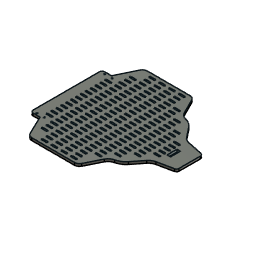
Electronics plate v13 (Autodesk Fusion 360 design; units mm, degrees)
Autodesk Fusion 360 part; units mm, degrees
(part 1 of 4)
sketch "Sketch2" plane through (0, 0, 0) normal (0, 1, 0) x (1, 0, 0)
  line L0 (-228.4396, 191.0218) -> (-250, 146.0218)
  line L1 (-249.9865, 0) -> (-228.4396, -44.9718)
  line L2 (-128.4396, 191.0218) -> (-228.4396, 191.0218)
  line L3 (-228.4396, -44.9718) -> (-128.4396, -44.9718)
  line L4 (-105.9194, 146.05) -> (-128.4396, 191.0218)
  line L5 (-128.4396, -44.9718) -> (-105.9194, 0)
  line L6 (-138.6977, 71.525) -> (-143.6977, 71.525)
  line L7 (-148.6977, 74.525) -> (-138.6977, 74.525)
  arc A0 (-138.6977, 71.525) -> (-138.6977, 74.525) centre (-138.6977, 73.025) ccw
  arc A1 (-148.6977, 74.525) -> (-148.6977, 71.525) centre (-148.6977, 73.025) ccw
  line L8 (-148.6977, 71.525) -> (-143.6977, 71.525)
  arc A2 (-208.6977, -35.475) -> (-208.6977, -38.475) centre (-208.6977, -36.975) ccw
  arc A3 (-198.6977, -38.475) -> (-198.6977, -35.475) centre (-198.6977, -36.975) ccw
  line L9 (-208.6977, -35.475) -> (-198.6977, -35.475)
  line L10 (-208.6977, -38.475) -> (-203.6977, -38.475)
  line L11 (-198.6977, -38.475) -> (-203.6977, -38.475)
  arc A4 (-188.6977, -35.475) -> (-188.6977, -38.475) centre (-188.6977, -36.975) ccw
  arc A5 (-178.6977, -38.475) -> (-178.6977, -35.475) centre (-178.6977, -36.975) ccw
  line L12 (-188.6977, -35.475) -> (-178.6977, -35.475)
  line L13 (-188.6977, -38.475) -> (-183.6977, -38.475)
  line L14 (-178.6977, -38.475) -> (-183.6977, -38.475)
  arc A6 (-168.6977, -35.475) -> (-168.6977, -38.475) centre (-168.6977, -36.975) ccw
  arc A7 (-158.6977, -38.475) -> (-158.6977, -35.475) centre (-158.6977, -36.975) ccw
  line L15 (-168.6977, -35.475) -> (-158.6977, -35.475)
  line L16 (-168.6977, -38.475) -> (-163.6977, -38.475)
  line L17 (-158.6977, -38.475) -> (-163.6977, -38.475)
  arc A8 (-148.6977, -35.475) -> (-148.6977, -38.475) centre (-148.6977, -36.975) ccw
  arc A9 (-138.6977, -38.475) -> (-138.6977, -35.475) centre (-138.6977, -36.975) ccw
  line L18 (-148.6977, -35.475) -> (-138.6977, -35.475)
  line L19 (-148.6977, -38.475) -> (-143.6977, -38.475)
  line L20 (-138.6977, -38.475) -> (-143.6977, -38.475)
  arc A10 (-208.6977, -25.475) -> (-208.6977, -28.475) centre (-208.6977, -26.975) ccw
  arc A11 (-198.6977, -28.475) -> (-198.6977, -25.475) centre (-198.6977, -26.975) ccw
  line L21 (-208.6977, -25.475) -> (-198.6977, -25.475)
  line L22 (-208.6977, -28.475) -> (-203.6977, -28.475)
  line L23 (-198.6977, -28.475) -> (-203.6977, -28.475)
  arc A12 (-188.6977, -25.475) -> (-188.6977, -28.475) centre (-188.6977, -26.975) ccw
  arc A13 (-178.6977, -28.475) -> (-178.6977, -25.475) centre (-178.6977, -26.975) ccw
  line L24 (-188.6977, -25.475) -> (-178.6977, -25.475)
  line L25 (-188.6977, -28.475) -> (-183.6977, -28.475)
  line L26 (-178.6977, -28.475) -> (-183.6977, -28.475)
  arc A14 (-168.6977, -25.475) -> (-168.6977, -28.475) centre (-168.6977, -26.975) ccw
  arc A15 (-158.6977, -28.475) -> (-158.6977, -25.475) centre (-158.6977, -26.975) ccw
  line L27 (-168.6977, -25.475) -> (-158.6977, -25.475)
  line L28 (-168.6977, -28.475) -> (-163.6977, -28.475)
  line L29 (-158.6977, -28.475) -> (-163.6977, -28.475)
  arc A16 (-148.6977, -25.475) -> (-148.6977, -28.475) centre (-148.6977, -26.975) ccw
  arc A17 (-138.6977, -28.475) -> (-138.6977, -25.475) centre (-138.6977, -26.975) ccw
  line L30 (-148.6977, -25.475) -> (-138.6977, -25.475)
  line L31 (-148.6977, -28.475) -> (-143.6977, -28.475)
  line L32 (-138.6977, -28.475) -> (-143.6977, -28.475)
  arc A18 (-228.6977, -15.475) -> (-228.6977, -18.475) centre (-228.6977, -16.975) ccw
  arc A19 (-218.6977, -18.475) -> (-218.6977, -15.475) centre (-218.6977, -16.975) ccw
  line L33 (-228.6977, -15.475) -> (-218.6977, -15.475)
  line L34 (-228.6977, -18.475) -> (-223.6977, -18.475)
  line L35 (-218.6977, -18.475) -> (-223.6977, -18.475)
  arc A20 (-208.6977, -15.475) -> (-208.6977, -18.475) centre (-208.6977, -16.975) ccw
  arc A21 (-198.6977, -18.475) -> (-198.6977, -15.475) centre (-198.6977, -16.975) ccw
  line L36 (-208.6977, -15.475) -> (-198.6977, -15.475)
  line L37 (-208.6977, -18.475) -> (-203.6977, -18.475)
  line L38 (-198.6977, -18.475) -> (-203.6977, -18.475)
  arc A22 (-188.6977, -15.475) -> (-188.6977, -18.475) centre (-188.6977, -16.975) ccw
  arc A23 (-178.6977, -18.475) -> (-178.6977, -15.475) centre (-178.6977, -16.975) ccw
  line L39 (-188.6977, -15.475) -> (-178.6977, -15.475)
  line L40 (-188.6977, -18.475) -> (-183.6977, -18.475)
  line L41 (-178.6977, -18.475) -> (-183.6977, -18.475)
  arc A24 (-168.6977, -15.475) -> (-168.6977, -18.475) centre (-168.6977, -16.975) ccw
  arc A25 (-158.6977, -18.475) -> (-158.6977, -15.475) centre (-158.6977, -16.975) ccw
  line L42 (-168.6977, -15.475) -> (-158.6977, -15.475)
  line L43 (-168.6977, -18.475) -> (-163.6977, -18.475)
  line L44 (-158.6977, -18.475) -> (-163.6977, -18.475)
  arc A26 (-148.6977, -15.475) -> (-148.6977, -18.475) centre (-148.6977, -16.975) ccw
  arc A27 (-138.6977, -18.475) -> (-138.6977, -15.475) centre (-138.6977, -16.975) ccw
  line L45 (-148.6977, -15.475) -> (-138.6977, -15.475)
  line L46 (-148.6977, -18.475) -> (-143.6977, -18.475)
  line L47 (-138.6977, -18.475) -> (-143.6977, -18.475)
  arc A28 (-228.6977, -5.475) -> (-228.6977, -8.475) centre (-228.6977, -6.975) ccw
  arc A29 (-218.6977, -8.475) -> (-218.6977, -5.475) centre (-218.6977, -6.975) ccw
  line L48 (-228.6977, -5.475) -> (-218.6977, -5.475)
  line L49 (-228.6977, -8.475) -> (-223.6977, -8.475)
  line L50 (-218.6977, -8.475) -> (-223.6977, -8.475)
  arc A30 (-208.6977, -5.475) -> (-208.6977, -8.475) centre (-208.6977, -6.975) ccw
  arc A31 (-198.6977, -8.475) -> (-198.6977, -5.475) centre (-198.6977, -6.975) ccw
  line L51 (-208.6977, -5.475) -> (-198.6977, -5.475)
  line L52 (-208.6977, -8.475) -> (-203.6977, -8.475)
  line L53 (-198.6977, -8.475) -> (-203.6977, -8.475)
  arc A32 (-188.6977, -5.475) -> (-188.6977, -8.475) centre (-188.6977, -6.975) ccw
  arc A33 (-178.6977, -8.475) -> (-178.6977, -5.475) centre (-178.6977, -6.975) ccw
  line L54 (-188.6977, -5.475) -> (-178.6977, -5.475)
  line L55 (-188.6977, -8.475) -> (-183.6977, -8.475)
  line L56 (-178.6977, -8.475) -> (-183.6977, -8.475)
  arc A34 (-168.6977, -5.475) -> (-168.6977, -8.475) centre (-168.6977, -6.975) ccw
  arc A35 (-158.6977, -8.475) -> (-158.6977, -5.475) centre (-158.6977, -6.975) ccw
  line L57 (-168.6977, -5.475) -> (-158.6977, -5.475)
  line L58 (-168.6977, -8.475) -> (-163.6977, -8.475)
  line L59 (-158.6977, -8.475) -> (-163.6977, -8.475)
  arc A36 (-148.6977, -5.475) -> (-148.6977, -8.475) centre (-148.6977, -6.975) ccw
  arc A37 (-138.6977, -8.475) -> (-138.6977, -5.475) centre (-138.6977, -6.975) ccw
  line L60 (-148.6977, -5.475) -> (-138.6977, -5.475)
  line L61 (-148.6977, -8.475) -> (-143.6977, -8.475)
  line L62 (-138.6977, -8.475) -> (-143.6977, -8.475)
  arc A38 (-128.6977, -5.475) -> (-128.6977, -8.475) centre (-128.6977, -6.975) ccw
  arc A39 (-118.6977, -8.475) -> (-118.6977, -5.475) centre (-118.6977, -6.975) ccw
  line L63 (-128.6977, -5.475) -> (-118.6977, -5.475)
  line L64 (-128.6977, -8.475) -> (-123.6977, -8.475)
  line L65 (-118.6977, -8.475) -> (-123.6977, -8.475)
  arc A40 (-228.6977, 4.525) -> (-228.6977, 1.525) centre (-228.6977, 3.025) ccw
  arc A41 (-218.6977, 1.525) -> (-218.6977, 4.525) centre (-218.6977, 3.025) ccw
  line L66 (-228.6977, 4.525) -> (-218.6977, 4.525)
  line L67 (-228.6977, 1.525) -> (-223.6977, 1.525)
  line L68 (-218.6977, 1.525) -> (-223.6977, 1.525)
  arc A42 (-208.6977, 4.525) -> (-208.6977, 1.525) centre (-208.6977, 3.025) ccw
  arc A43 (-198.6977, 1.525) -> (-198.6977, 4.525) centre (-198.6977, 3.025) ccw
  line L69 (-208.6977, 4.525) -> (-198.6977, 4.525)
  line L70 (-208.6977, 1.525) -> (-203.6977, 1.525)
  line L71 (-198.6977, 1.525) -> (-203.6977, 1.525)
  arc A44 (-188.6977, 4.525) -> (-188.6977, 1.525) centre (-188.6977, 3.025) ccw
  arc A45 (-178.6977, 1.525) -> (-178.6977, 4.525) centre (-178.6977, 3.025) ccw
  line L72 (-188.6977, 4.525) -> (-178.6977, 4.525)
  line L73 (-188.6977, 1.525) -> (-183.6977, 1.525)
  line L74 (-178.6977, 1.525) -> (-183.6977, 1.525)
  arc A46 (-168.6977, 4.525) -> (-168.6977, 1.525) centre (-168.6977, 3.025) ccw
  arc A47 (-158.6977, 1.525) -> (-158.6977, 4.525) centre (-158.6977, 3.025) ccw
  line L75 (-168.6977, 4.525) -> (-158.6977, 4.525)
  line L76 (-168.6977, 1.525) -> (-163.6977, 1.525)
  line L77 (-158.6977, 1.525) -> (-163.6977, 1.525)
  arc A48 (-148.6977, 4.525) -> (-148.6977, 1.525) centre (-148.6977, 3.025) ccw
  arc A49 (-138.6977, 1.525) -> (-138.6977, 4.525) centre (-138.6977, 3.025) ccw
  line L78 (-148.6977, 4.525) -> (-138.6977, 4.525)
  line L79 (-148.6977, 1.525) -> (-143.6977, 1.525)
  line L80 (-138.6977, 1.525) -> (-143.6977, 1.525)
  arc A50 (-128.6977, 4.525) -> (-128.6977, 1.525) centre (-128.6977, 3.025) ccw
  arc A51 (-118.6977, 1.525) -> (-118.6977, 4.525) centre (-118.6977, 3.025) ccw
  line L81 (-128.6977, 4.525) -> (-118.6977, 4.525)
  line L82 (-128.6977, 1.525) -> (-123.6977, 1.525)
  line L83 (-118.6977, 1.525) -> (-123.6977, 1.525)
  arc A52 (-248.6977, 14.525) -> (-248.6977, 11.525) centre (-248.6977, 13.025) ccw
  arc A53 (-238.6977, 11.525) -> (-238.6977, 14.525) centre (-238.6977, 13.025) ccw
  line L84 (-248.6977, 14.525) -> (-238.6977, 14.525)
  line L85 (-248.6977, 11.525) -> (-243.6977, 11.525)
  line L86 (-238.6977, 11.525) -> (-243.6977, 11.525)
  arc A54 (-228.6977, 14.525) -> (-228.6977, 11.525) centre (-228.6977, 13.025) ccw
  arc A55 (-218.6977, 11.525) -> (-218.6977, 14.525) centre (-218.6977, 13.025) ccw
  line L87 (-228.6977, 14.525) -> (-218.6977, 14.525)
  line L88 (-228.6977, 11.525) -> (-223.6977, 11.525)
  line L89 (-218.6977, 11.525) -> (-223.6977, 11.525)
  arc A56 (-208.6977, 14.525) -> (-208.6977, 11.525) centre (-208.6977, 13.025) ccw
  arc A57 (-198.6977, 11.525) -> (-198.6977, 14.525) centre (-198.6977, 13.025) ccw
  line L90 (-208.6977, 14.525) -> (-198.6977, 14.525)
  line L91 (-208.6977, 11.525) -> (-203.6977, 11.525)
  line L92 (-198.6977, 11.525) -> (-203.6977, 11.525)
  arc A58 (-188.6977, 14.525) -> (-188.6977, 11.525) centre (-188.6977, 13.025) ccw
  arc A59 (-178.6977, 11.525) -> (-178.6977, 14.525) centre (-178.6977, 13.025) ccw
  line L93 (-188.6977, 14.525) -> (-178.6977, 14.525)
  line L94 (-188.6977, 11.525) -> (-183.6977, 11.525)
  line L95 (-178.6977, 11.525) -> (-183.6977, 11.525)
  arc A60 (-168.6977, 14.525) -> (-168.6977, 11.525) centre (-168.6977, 13.025) ccw
  arc A61 (-158.6977, 11.525) -> (-158.6977, 14.525) centre (-158.6977, 13.025) ccw
  line L96 (-168.6977, 14.525) -> (-158.6977, 14.525)
  line L97 (-168.6977, 11.525) -> (-163.6977, 11.525)
  line L98 (-158.6977, 11.525) -> (-163.6977, 11.525)
  arc A62 (-148.6977, 14.525) -> (-148.6977, 11.525) centre (-148.6977, 13.025) ccw
  arc A63 (-138.6977, 11.525) -> (-138.6977, 14.525) centre (-138.6977, 13.025) ccw
  line L99 (-148.6977, 14.525) -> (-138.6977, 14.525)
  line L100 (-148.6977, 11.525) -> (-143.6977, 11.525)
  line L101 (-138.6977, 11.525) -> (-143.6977, 11.525)
  arc A64 (-128.6977, 14.525) -> (-128.6977, 11.525) centre (-128.6977, 13.025) ccw
  arc A65 (-118.6977, 11.525) -> (-118.6977, 14.525) centre (-118.6977, 13.025) ccw
  line L102 (-128.6977, 14.525) -> (-118.6977, 14.525)
  line L103 (-128.6977, 11.525) -> (-123.6977, 11.525)
  line L104 (-118.6977, 11.525) -> (-123.6977, 11.525)
  arc A66 (-108.6977, 14.525) -> (-108.6977, 11.525) centre (-108.6977, 13.025) ccw
  arc A67 (-98.6977, 11.525) -> (-98.6977, 14.525) centre (-98.6977, 13.025) ccw
  line L105 (-108.6977, 14.525) -> (-98.6977, 14.525)
  line L106 (-108.6977, 11.525) -> (-103.6977, 11.525)
  line L107 (-98.6977, 11.525) -> (-103.6977, 11.525)
  arc A68 (-248.6977, 24.525) -> (-248.6977, 21.525) centre (-248.6977, 23.025) ccw
  arc A69 (-238.6977, 21.525) -> (-238.6977, 24.525) centre (-238.6977, 23.025) ccw
  line L108 (-248.6977, 24.525) -> (-238.6977, 24.525)
  line L109 (-248.6977, 21.525) -> (-243.6977, 21.525)
  line L110 (-238.6977, 21.525) -> (-243.6977, 21.525)
  arc A70 (-228.6977, 24.525) -> (-228.6977, 21.525) centre (-228.6977, 23.025) ccw
  arc A71 (-218.6977, 21.525) -> (-218.6977, 24.525) centre (-218.6977, 23.025) ccw
  line L111 (-228.6977, 24.525) -> (-218.6977, 24.525)
  line L112 (-228.6977, 21.525) -> (-223.6977, 21.525)
  line L113 (-218.6977, 21.525) -> (-223.6977, 21.525)
  arc A72 (-208.6977, 24.525) -> (-208.6977, 21.525) centre (-208.6977, 23.025) ccw
  arc A73 (-198.6977, 21.525) -> (-198.6977, 24.525) centre (-198.6977, 23.025) ccw
  line L114 (-208.6977, 24.525) -> (-198.6977, 24.525)
  line L115 (-208.6977, 21.525) -> (-203.6977, 21.525)
  line L116 (-198.6977, 21.525) -> (-203.6977, 21.525)
  arc A74 (-188.6977, 24.525) -> (-188.6977, 21.525) centre (-188.6977, 23.025) ccw
  arc A75 (-178.6977, 21.525) -> (-178.6977, 24.525) centre (-178.6977, 23.025) ccw
  line L117 (-188.6977, 24.525) -> (-178.6977, 24.525)
  line L118 (-188.6977, 21.525) -> (-183.6977, 21.525)
  line L119 (-178.6977, 21.525) -> (-183.6977, 21.525)
  arc A76 (-168.6977, 24.525) -> (-168.6977, 21.525) centre (-168.6977, 23.025) ccw
  arc A77 (-158.6977, 21.525) -> (-158.6977, 24.525) centre (-158.6977, 23.025) ccw
  line L120 (-168.6977, 24.525) -> (-158.6977, 24.525)
  line L121 (-168.6977, 21.525) -> (-163.6977, 21.525)
  line L122 (-158.6977, 21.525) -> (-163.6977, 21.525)
  arc A78 (-148.6977, 24.525) -> (-148.6977, 21.525) centre (-148.6977, 23.025) ccw
  arc A79 (-138.6977, 21.525) -> (-138.6977, 24.525) centre (-138.6977, 23.025) ccw
  line L123 (-148.6977, 24.525) -> (-138.6977, 24.525)
  line L124 (-148.6977, 21.525) -> (-143.6977, 21.525)
  line L125 (-138.6977, 21.525) -> (-143.6977, 21.525)
  arc A80 (-128.6977, 24.525) -> (-128.6977, 21.525) centre (-128.6977, 23.025) ccw
  arc A81 (-118.6977, 21.525) -> (-118.6977, 24.525) centre (-118.6977, 23.025) ccw
  line L126 (-128.6977, 24.525) -> (-118.6977, 24.525)
  line L127 (-128.6977, 21.525) -> (-123.6977, 21.525)
  line L128 (-118.6977, 21.525) -> (-123.6977, 21.525)
  arc A82 (-108.6977, 24.525) -> (-108.6977, 21.525) centre (-108.6977, 23.025) ccw
  arc A83 (-98.6977, 21.525) -> (-98.6977, 24.525) centre (-98.6977, 23.025) ccw
  line L129 (-108.6977, 24.525) -> (-98.6977, 24.525)
  line L130 (-108.6977, 21.525) -> (-103.6977, 21.525)
  line L131 (-98.6977, 21.525) -> (-103.6977, 21.525)
  arc A84 (-248.6977, 34.525) -> (-248.6977, 31.525) centre (-248.6977, 33.025) ccw
  arc A85 (-238.6977, 31.525) -> (-238.6977, 34.525) centre (-238.6977, 33.025) ccw
  line L132 (-248.6977, 34.525) -> (-238.6977, 34.525)
  line L133 (-248.6977, 31.525) -> (-243.6977, 31.525)
  line L134 (-238.6977, 31.525) -> (-243.6977, 31.525)
  arc A86 (-228.6977, 34.525) -> (-228.6977, 31.525) centre (-228.6977, 33.025) ccw
  arc A87 (-218.6977, 31.525) -> (-218.6977, 34.525) centre (-218.6977, 33.025) ccw
  line L135 (-228.6977, 34.525) -> (-218.6977, 34.525)
  line L136 (-228.6977, 31.525) -> (-223.6977, 31.525)
  line L137 (-218.6977, 31.525) -> (-223.6977, 31.525)
  arc A88 (-208.6977, 34.525) -> (-208.6977, 31.525) centre (-208.6977, 33.025) ccw
  arc A89 (-198.6977, 31.525) -> (-198.6977, 34.525) centre (-198.6977, 33.025) ccw
  line L138 (-208.6977, 34.525) -> (-198.6977, 34.525)
  line L139 (-208.6977, 31.525) -> (-203.6977, 31.525)
  line L140 (-198.6977, 31.525) -> (-203.6977, 31.525)
  arc A90 (-188.6977, 34.525) -> (-188.6977, 31.525) centre (-188.6977, 33.025) ccw
  arc A91 (-178.6977, 31.525) -> (-178.6977, 34.525) centre (-178.6977, 33.025) ccw
  line L141 (-188.6977, 34.525) -> (-178.6977, 34.525)
  line L142 (-188.6977, 31.525) -> (-183.6977, 31.525)
  line L143 (-178.6977, 31.525) -> (-183.6977, 31.525)
  arc A92 (-168.6977, 34.525) -> (-168.6977, 31.525) centre (-168.6977, 33.025) ccw
  arc A93 (-158.6977, 31.525) -> (-158.6977, 34.525) centre (-158.6977, 33.025) ccw
  line L144 (-168.6977, 34.525) -> (-158.6977, 34.525)
  line L145 (-168.6977, 31.525) -> (-163.6977, 31.525)
  line L146 (-158.6977, 31.525) -> (-163.6977, 31.525)
  arc A94 (-148.6977, 34.525) -> (-148.6977, 31.525) centre (-148.6977, 33.025) ccw
  arc A95 (-138.6977, 31.525) -> (-138.6977, 34.525) centre (-138.6977, 33.025) ccw
  line L147 (-148.6977, 34.525) -> (-138.6977, 34.525)
  line L148 (-148.6977, 31.525) -> (-143.6977, 31.525)
  line L149 (-138.6977, 31.525) -> (-143.6977, 31.525)
  arc A96 (-128.6977, 34.525) -> (-128.6977, 31.525) centre (-128.6977, 33.025) ccw
  arc A97 (-118.6977, 31.525) -> (-118.6977, 34.525) centre (-118.6977, 33.025) ccw
  line L150 (-128.6977, 34.525) -> (-118.6977, 34.525)
  line L151 (-128.6977, 31.525) -> (-123.6977, 31.525)
  line L152 (-118.6977, 31.525) -> (-123.6977, 31.525)
  arc A98 (-108.6977, 34.525) -> (-108.6977, 31.525) centre (-108.6977, 33.025) ccw
  arc A99 (-98.6977, 31.525) -> (-98.6977, 34.525) centre (-98.6977, 33.025) ccw
  line L153 (-108.6977, 34.525) -> (-98.6977, 34.525)
  line L154 (-108.6977, 31.525) -> (-103.6977, 31.525)
  line L155 (-98.6977, 31.525) -> (-103.6977, 31.525)
  arc A100 (-88.6977, 34.525) -> (-88.6977, 31.525) centre (-88.6977, 33.025) ccw
  arc A101 (-78.6977, 31.525) -> (-78.6977, 34.525) centre (-78.6977, 33.025) ccw
  line L156 (-88.6977, 34.525) -> (-78.6977, 34.525)
  line L157 (-88.6977, 31.525) -> (-83.6977, 31.525)
  line L158 (-78.6977, 31.525) -> (-83.6977, 31.525)
  arc A102 (-248.6977, 44.525) -> (-248.6977, 41.525) centre (-248.6977, 43.025) ccw
  arc A103 (-238.6977, 41.525) -> (-238.6977, 44.525) centre (-238.6977, 43.025) ccw
  line L159 (-248.6977, 44.525) -> (-238.6977, 44.525)
  line L160 (-248.6977, 41.525) -> (-243.6977, 41.525)
  line L161 (-238.6977, 41.525) -> (-243.6977, 41.525)
  arc A104 (-228.6977, 44.525) -> (-228.6977, 41.525) centre (-228.6977, 43.025) ccw
  arc A105 (-218.6977, 41.525) -> (-218.6977, 44.525) centre (-218.6977, 43.025) ccw
  line L162 (-228.6977, 44.525) -> (-218.6977, 44.525)
  line L163 (-228.6977, 41.525) -> (-223.6977, 41.525)
  line L164 (-218.6977, 41.525) -> (-223.6977, 41.525)
  arc A106 (-208.6977, 44.525) -> (-208.6977, 41.525) centre (-208.6977, 43.025) ccw
  arc A107 (-198.6977, 41.525) -> (-198.6977, 44.525) centre (-198.6977, 43.025) ccw
  line L165 (-208.6977, 44.525) -> (-198.6977, 44.525)
  line L166 (-208.6977, 41.525) -> (-203.6977, 41.525)
  line L167 (-198.6977, 41.525) -> (-203.6977, 41.525)
  arc A108 (-188.6977, 44.525) -> (-188.6977, 41.525) centre (-188.6977, 43.025) ccw
  arc A109 (-178.6977, 41.525) -> (-178.6977, 44.525) centre (-178.6977, 43.025) ccw
  line L168 (-188.6977, 44.525) -> (-178.6977, 44.525)
  line L169 (-188.6977, 41.525) -> (-183.6977, 41.525)
  line L170 (-178.6977, 41.525) -> (-183.6977, 41.525)
  arc A110 (-168.6977, 44.525) -> (-168.6977, 41.525) centre (-168.6977, 43.025) ccw
  arc A111 (-158.6977, 41.525) -> (-158.6977, 44.525) centre (-158.6977, 43.025) ccw
  line L171 (-168.6977, 44.525) -> (-158.6977, 44.525)
  line L172 (-168.6977, 41.525) -> (-163.6977, 41.525)
  line L173 (-158.6977, 41.525) -> (-163.6977, 41.525)
  arc A112 (-148.6977, 44.525) -> (-148.6977, 41.525) centre (-148.6977, 43.025) ccw
  arc A113 (-138.6977, 41.525) -> (-138.6977, 44.525) centre (-138.6977, 43.025) ccw
  line L174 (-148.6977, 44.525) -> (-138.6977, 44.525)
  line L175 (-148.6977, 41.525) -> (-143.6977, 41.525)
  line L176 (-138.6977, 41.525) -> (-143.6977, 41.525)
  arc A114 (-128.6977, 44.525) -> (-128.6977, 41.525) centre (-128.6977, 43.025) ccw
  arc A115 (-118.6977, 41.525) -> (-118.6977, 44.525) centre (-118.6977, 43.025) ccw
  line L177 (-128.6977, 44.525) -> (-118.6977, 44.525)
  line L178 (-128.6977, 41.525) -> (-123.6977, 41.525)
  line L179 (-118.6977, 41.525) -> (-123.6977, 41.525)
  arc A116 (-108.6977, 44.525) -> (-108.6977, 41.525) centre (-108.6977, 43.025) ccw
  arc A117 (-98.6977, 41.525) -> (-98.6977, 44.525) centre (-98.6977, 43.025) ccw
  line L180 (-108.6977, 44.525) -> (-98.6977, 44.525)
  line L181 (-108.6977, 41.525) -> (-103.6977, 41.525)
  line L182 (-98.6977, 41.525) -> (-103.6977, 41.525)
  arc A118 (-88.6977, 44.525) -> (-88.6977, 41.525) centre (-88.6977, 43.025) ccw
  arc A119 (-78.6977, 41.525) -> (-78.6977, 44.525) centre (-78.6977, 43.025) ccw
  line L183 (-88.6977, 44.525) -> (-78.6977, 44.525)
  line L184 (-88.6977, 41.525) -> (-83.6977, 41.525)
  line L185 (-78.6977, 41.525) -> (-83.6977, 41.525)
  arc A120 (-248.6977, 54.525) -> (-248.6977, 51.525) centre (-248.6977, 53.025) ccw
  arc A121 (-238.6977, 51.525) -> (-238.6977, 54.525) centre (-238.6977, 53.025) ccw
  line L186 (-248.6977, 54.525) -> (-238.6977, 54.525)
  line L187 (-248.6977, 51.525) -> (-243.6977, 51.525)
  line L188 (-238.6977, 51.525) -> (-243.6977, 51.525)
  arc A122 (-228.6977, 54.525) -> (-228.6977, 51.525) centre (-228.6977, 53.025) ccw
  arc A123 (-218.6977, 51.525) -> (-218.6977, 54.525) centre (-218.6977, 53.025) ccw
  line L189 (-228.6977, 54.525) -> (-218.6977, 54.525)
  line L190 (-228.6977, 51.525) -> (-223.6977, 51.525)
  line L191 (-218.6977, 51.525) -> (-223.6977, 51.525)
  arc A124 (-208.6977, 54.525) -> (-208.6977, 51.525) centre (-208.6977, 53.025) ccw
  arc A125 (-198.6977, 51.525) -> (-198.6977, 54.525) centre (-198.6977, 53.025) ccw
  line L192 (-208.6977, 54.525) -> (-198.6977, 54.525)
  line L193 (-208.6977, 51.525) -> (-203.6977, 51.525)
  line L194 (-198.6977, 51.525) -> (-203.6977, 51.525)
  arc A126 (-188.6977, 54.525) -> (-188.6977, 51.525) centre (-188.6977, 53.025) ccw
  arc A127 (-178.6977, 51.525) -> (-178.6977, 54.525) centre (-178.6977, 53.025) ccw
  line L195 (-188.6977, 54.525) -> (-178.6977, 54.525)
  line L196 (-188.6977, 51.525) -> (-183.6977, 51.525)
  line L197 (-178.6977, 51.525) -> (-183.6977, 51.525)
  arc A128 (-168.6977, 54.525) -> (-168.6977, 51.525) centre (-168.6977, 53.025) ccw
  arc A129 (-158.6977, 51.525) -> (-158.6977, 54.525) centre (-158.6977, 53.025) ccw
  line L198 (-168.6977, 54.525) -> (-158.6977, 54.525)
  line L199 (-168.6977, 51.525) -> (-163.6977, 51.525)
  line L200 (-158.6977, 51.525) -> (-163.6977, 51.525)
  arc A130 (-148.6977, 54.525) -> (-148.6977, 51.525) centre (-148.6977, 53.025) ccw
  arc A131 (-138.6977, 51.525) -> (-138.6977, 54.525) centre (-138.6977, 53.025) ccw
  line L201 (-148.6977, 54.525) -> (-138.6977, 54.525)
  line L202 (-148.6977, 51.525) -> (-143.6977, 51.525)
  line L203 (-138.6977, 51.525) -> (-143.6977, 51.525)
  arc A132 (-128.6977, 54.525) -> (-128.6977, 51.525) centre (-128.6977, 53.025) ccw
  arc A133 (-118.6977, 51.525) -> (-118.6977, 54.525) centre (-118.6977, 53.025) ccw
  line L204 (-128.6977, 54.525) -> (-118.6977, 54.525)
  line L205 (-128.6977, 51.525) -> (-123.6977, 51.525)
  line L206 (-118.6977, 51.525) -> (-123.6977, 51.525)
  arc A134 (-108.6977, 54.525) -> (-108.6977, 51.525) centre (-108.6977, 53.025) ccw
  arc A135 (-98.6977, 51.525) -> (-98.6977, 54.525) centre (-98.6977, 53.025) ccw
  line L207 (-108.6977, 54.525) -> (-98.6977, 54.525)
  line L208 (-108.6977, 51.525) -> (-103.6977, 51.525)
  line L209 (-98.6977, 51.525) -> (-103.6977, 51.525)
  arc A136 (-88.6977, 54.525) -> (-88.6977, 51.525) centre (-88.6977, 53.025) ccw
  arc A137 (-78.6977, 51.525) -> (-78.6977, 54.525) centre (-78.6977, 53.025) ccw
  line L210 (-88.6977, 54.525) -> (-78.6977, 54.525)
  line L211 (-88.6977, 51.525) -> (-83.6977, 51.525)
  line L212 (-78.6977, 51.525) -> (-83.6977, 51.525)
  arc A138 (-68.6977, 54.525) -> (-68.6977, 51.525) centre (-68.6977, 53.025) ccw
  arc A139 (-58.6977, 51.525) -> (-58.6977, 54.525) centre (-58.6977, 53.025) ccw
  line L213 (-68.6977, 54.525) -> (-58.6977, 54.525)
  line L214 (-68.6977, 51.525) -> (-63.6977, 51.525)
  line L215 (-58.6977, 51.525) -> (-63.6977, 51.525)
  arc A140 (-248.6977, 64.525) -> (-248.6977, 61.525) centre (-248.6977, 63.025) ccw
  arc A141 (-238.6977, 61.525) -> (-238.6977, 64.525) centre (-238.6977, 63.025) ccw
  line L216 (-248.6977, 64.525) -> (-238.6977, 64.525)
  line L217 (-248.6977, 61.525) -> (-243.6977, 61.525)
  line L218 (-238.6977, 61.525) -> (-243.6977, 61.525)
  arc A142 (-228.6977, 64.525) -> (-228.6977, 61.525) centre (-228.6977, 63.025) ccw
  arc A143 (-218.6977, 61.525) -> (-218.6977, 64.525) centre (-218.6977, 63.025) ccw
  line L219 (-228.6977, 64.525) -> (-218.6977, 64.525)
  line L220 (-228.6977, 61.525) -> (-223.6977, 61.525)
  line L221 (-218.6977, 61.525) -> (-223.6977, 61.525)
  arc A144 (-208.6977, 64.525) -> (-208.6977, 61.525) centre (-208.6977, 63.025) ccw
  arc A145 (-198.6977, 61.525) -> (-198.6977, 64.525) centre (-198.6977, 63.025) ccw
  line L222 (-208.6977, 64.525) -> (-198.6977, 64.525)
  line L223 (-208.6977, 61.525) -> (-203.6977, 61.525)
  line L224 (-198.6977, 61.525) -> (-203.6977, 61.525)
  arc A146 (-188.6977, 64.525) -> (-188.6977, 61.525) centre (-188.6977, 63.025) ccw
  arc A147 (-178.6977, 61.525) -> (-178.6977, 64.525) centre (-178.6977, 63.025) ccw
  line L225 (-188.6977, 64.525) -> (-178.6977, 64.525)
  line L226 (-188.6977, 61.525) -> (-183.6977, 61.525)
  line L227 (-178.6977, 61.525) -> (-183.6977, 61.525)
  arc A148 (-168.6977, 64.525) -> (-168.6977, 61.525) centre (-168.6977, 63.025) ccw
  arc A149 (-158.6977, 61.525) -> (-158.6977, 64.525) centre (-158.6977, 63.025) ccw
  line L228 (-168.6977, 64.525) -> (-158.6977, 64.525)
  line L229 (-168.6977, 61.525) -> (-163.6977, 61.525)
  line L230 (-158.6977, 61.525) -> (-163.6977, 61.525)
  arc A150 (-148.6977, 64.525) -> (-148.6977, 61.525) centre (-148.6977, 63.025) ccw
  arc A151 (-138.6977, 61.525) -> (-138.6977, 64.525) centre (-138.6977, 63.025) ccw
  line L231 (-148.6977, 64.525) -> (-138.6977, 64.525)
  line L232 (-148.6977, 61.525) -> (-143.6977, 61.525)
  line L233 (-138.6977, 61.525) -> (-143.6977, 61.525)
  arc A152 (-128.6977, 64.525) -> (-128.6977, 61.525) centre (-128.6977, 63.025) ccw
  arc A153 (-118.6977, 61.525) -> (-118.6977, 64.525) centre (-118.6977, 63.025) ccw
  line L234 (-128.6977, 64.525) -> (-118.6977, 64.525)
  line L235 (-128.6977, 61.525) -> (-123.6977, 61.525)
  line L236 (-118.6977, 61.525) -> (-123.6977, 61.525)
  arc A154 (-108.6977, 64.525) -> (-108.6977, 61.525) centre (-108.6977, 63.025) ccw
  arc A155 (-98.6977, 61.525) -> (-98.6977, 64.525) centre (-98.6977, 63.025) ccw
  line L237 (-108.6977, 64.525) -> (-98.6977, 64.525)
  line L238 (-108.6977, 61.525) -> (-103.6977, 61.525)
  line L239 (-98.6977, 61.525) -> (-103.6977, 61.525)
  arc A156 (-88.6977, 64.525) -> (-88.6977, 61.525) centre (-88.6977, 63.025) ccw
  arc A157 (-78.6977, 61.525) -> (-78.6977, 64.525) centre (-78.6977, 63.025) ccw
  line L240 (-88.6977, 64.525) -> (-78.6977, 64.525)
  line L241 (-88.6977, 61.525) -> (-83.6977, 61.525)
  line L242 (-78.6977, 61.525) -> (-83.6977, 61.525)
  arc A158 (-68.6977, 64.525) -> (-68.6977, 61.525) centre (-68.6977, 63.025) ccw
  arc A159 (-58.6977, 61.525) -> (-58.6977, 64.525) centre (-58.6977, 63.025) ccw
  line L243 (-68.6977, 64.525) -> (-58.6977, 64.525)
  line L244 (-68.6977, 61.525) -> (-63.6977, 61.525)
  line L245 (-58.6977, 61.525) -> (-63.6977, 61.525)
  arc A160 (-248.6977, 74.525) -> (-248.6977, 71.525) centre (-248.6977, 73.025) ccw
  arc A161 (-238.6977, 71.525) -> (-238.6977, 74.525) centre (-238.6977, 73.025) ccw
  line L246 (-248.6977, 74.525) -> (-238.6977, 74.525)
  line L247 (-248.6977, 71.525) -> (-243.6977, 71.525)
  line L248 (-238.6977, 71.525) -> (-243.6977, 71.525)
  arc A162 (-228.6977, 74.525) -> (-228.6977, 71.525) centre (-228.6977, 73.025) ccw
  arc A163 (-218.6977, 71.525) -> (-218.6977, 74.525) centre (-218.6977, 73.025) ccw
  line L249 (-228.6977, 74.525) -> (-218.6977, 74.525)
  line L250 (-228.6977, 71.525) -> (-223.6977, 71.525)
  line L251 (-218.6977, 71.525) -> (-223.6977, 71.525)
  arc A164 (-208.6977, 74.525) -> (-208.6977, 71.525) centre (-208.6977, 73.025) ccw
  arc A165 (-198.6977, 71.525) -> (-198.6977, 74.525) centre (-198.6977, 73.025) ccw
  line L252 (-208.6977, 74.525) -> (-198.6977, 74.525)
  line L253 (-208.6977, 71.525) -> (-203.6977, 71.525)
  line L254 (-198.6977, 71.525) -> (-203.6977, 71.525)
  arc A166 (-188.6977, 74.525) -> (-188.6977, 71.525) centre (-188.6977, 73.025) ccw
  arc A167 (-178.6977, 71.525) -> (-178.6977, 74.525) centre (-178.6977, 73.025) ccw
  line L255 (-188.6977, 74.525) -> (-178.6977, 74.525)
  line L256 (-188.6977, 71.525) -> (-183.6977, 71.525)
  line L257 (-178.6977, 71.525) -> (-183.6977, 71.525)
  arc A168 (-168.6977, 74.525) -> (-168.6977, 71.525) centre (-168.6977, 73.025) ccw
  arc A169 (-158.6977, 71.525) -> (-158.6977, 74.525) centre (-158.6977, 73.025) ccw
  line L258 (-168.6977, 74.525) -> (-158.6977, 74.525)
  line L259 (-168.6977, 71.525) -> (-163.6977, 71.525)
  line L260 (-158.6977, 71.525) -> (-163.6977, 71.525)
  arc A170 (-128.6977, 74.525) -> (-128.6977, 71.525) centre (-128.6977, 73.025) ccw
  arc A171 (-118.6977, 71.525) -> (-118.6977, 74.525) centre (-118.6977, 73.025) ccw
  line L261 (-128.6977, 74.525) -> (-118.6977, 74.525)
  line L262 (-128.6977, 71.525) -> (-123.6977, 71.525)
  line L263 (-118.6977, 71.525) -> (-123.6977, 71.525)
  arc A172 (-108.6977, 74.525) -> (-108.6977, 71.525) centre (-108.6977, 73.025) ccw
  arc A173 (-98.6977, 71.525) -> (-98.6977, 74.525) centre (-98.6977, 73.025) ccw
  line L264 (-108.6977, 74.525) -> (-98.6977, 74.525)
  line L265 (-108.6977, 71.525) -> (-103.6977, 71.525)
  line L266 (-98.6977, 71.525) -> (-103.6977, 71.525)
  arc A174 (-88.6977, 74.525) -> (-88.6977, 71.525) centre (-88.6977, 73.025) ccw
  arc A175 (-78.6977, 71.525) -> (-78.6977, 74.525) centre (-78.6977, 73.025) ccw
  line L267 (-88.6977, 74.525) -> (-78.6977, 74.525)
  line L268 (-88.6977, 71.525) -> (-83.6977, 71.525)
  line L269 (-78.6977, 71.525) -> (-83.6977, 71.525)
  arc A176 (-68.6977, 74.525) -> (-68.6977, 71.525) centre (-68.6977, 73.025) ccw
  arc A177 (-58.6977, 71.525) -> (-58.6977, 74.525) centre (-58.6977, 73.025) ccw
  line L270 (-68.6977, 74.525) -> (-58.6977, 74.525)
  line L271 (-68.6977, 71.525) -> (-63.6977, 71.525)
  line L272 (-58.6977, 71.525) -> (-63.6977, 71.525)
  arc A178 (-248.6977, 84.525) -> (-248.6977, 81.525) centre (-248.6977, 83.025) ccw
  arc A179 (-238.6977, 81.525) -> (-238.6977, 84.525) centre (-238.6977, 83.025) ccw
  line L273 (-248.6977, 84.525) -> (-238.6977, 84.525)
  line L274 (-248.6977, 81.525) -> (-243.6977, 81.525)
  line L275 (-238.6977, 81.525) -> (-243.6977, 81.525)
  arc A180 (-228.6977, 84.525) -> (-228.6977, 81.525) centre (-228.6977, 83.025) ccw
  arc A181 (-218.6977, 81.525) -> (-218.6977, 84.525) centre (-218.6977, 83.025) ccw
  line L276 (-228.6977, 84.525) -> (-218.6977, 84.525)
  line L277 (-228.6977, 81.525) -> (-223.6977, 81.525)
  line L278 (-218.6977, 81.525) -> (-223.6977, 81.525)
  arc A182 (-208.6977, 84.525) -> (-208.6977, 81.525) centre (-208.6977, 83.025) ccw
  arc A183 (-198.6977, 81.525) -> (-198.6977, 84.525) centre (-198.6977, 83.025) ccw
  line L279 (-208.6977, 84.525) -> (-198.6977, 84.525)
  line L280 (-208.6977, 81.525) -> (-203.6977, 81.525)
  line L281 (-198.6977, 81.525) -> (-203.6977, 81.525)
  arc A184 (-188.6977, 84.525) -> (-188.6977, 81.525) centre (-188.6977, 83.025) ccw
  arc A185 (-178.6977, 81.525) -> (-178.6977, 84.525) centre (-178.6977, 83.025) ccw
  line L282 (-188.6977, 84.525) -> (-178.6977, 84.525)
  line L283 (-188.6977, 81.525) -> (-183.6977, 81.525)
  line L284 (-178.6977, 81.525) -> (-183.6977, 81.525)
  arc A186 (-168.6977, 84.525) -> (-168.6977, 81.525) centre (-168.6977, 83.025) ccw
  arc A187 (-158.6977, 81.525) -> (-158.6977, 84.525) centre (-158.6977, 83.025) ccw
  line L285 (-168.6977, 84.525) -> (-158.6977, 84.525)
  line L286 (-168.6977, 81.525) -> (-163.6977, 81.525)
  line L287 (-158.6977, 81.525) -> (-163.6977, 81.525)
  arc A188 (-148.6977, 84.525) -> (-148.6977, 81.525) centre (-148.6977, 83.025) ccw
  arc A189 (-138.6977, 81.525) -> (-138.6977, 84.525) centre (-138.6977, 83.025) ccw
  line L288 (-148.6977, 84.525) -> (-138.6977, 84.525)
  line L289 (-148.6977, 81.525) -> (-143.6977, 81.525)
  line L290 (-138.6977, 81.525) -> (-143.6977, 81.525)
  arc A190 (-128.6977, 84.525) -> (-128.6977, 81.525) centre (-128.6977, 83.025) ccw
  arc A191 (-118.6977, 81.525) -> (-118.6977, 84.525) centre (-118.6977, 83.025) ccw
  line L291 (-128.6977, 84.525) -> (-118.6977, 84.525)
  line L292 (-128.6977, 81.525) -> (-123.6977, 81.525)
  line L293 (-118.6977, 81.525) -> (-123.6977, 81.525)
  arc A192 (-108.6977, 84.525) -> (-108.6977, 81.525) centre (-108.6977, 83.025) ccw
  arc A193 (-98.6977, 81.525) -> (-98.6977, 84.525) centre (-98.6977, 83.025) ccw
  line L294 (-108.6977, 84.525) -> (-98.6977, 84.525)
  line L295 (-108.6977, 81.525) -> (-103.6977, 81.525)
  line L296 (-98.6977, 81.525) -> (-103.6977, 81.525)
  arc A194 (-88.6977, 84.525) -> (-88.6977, 81.525) centre (-88.6977, 83.025) ccw
  arc A195 (-78.6977, 81.525) -> (-78.6977, 84.525) centre (-78.6977, 83.025) ccw
  line L297 (-88.6977, 84.525) -> (-78.6977, 84.525)
  line L298 (-88.6977, 81.525) -> (-83.6977, 81.525)
  line L299 (-78.6977, 81.525) -> (-83.6977, 81.525)
  arc A196 (-68.6977, 84.525) -> (-68.6977, 81.525) centre (-68.6977, 83.025) ccw
  arc A197 (-58.6977, 81.525) -> (-58.6977, 84.525) centre (-58.6977, 83.025) ccw
  line L300 (-68.6977, 84.525) -> (-58.6977, 84.525)
  line L301 (-68.6977, 81.525) -> (-63.6977, 81.525)
  line L302 (-58.6977, 81.525) -> (-63.6977, 81.525)
  arc A198 (-248.6977, 94.525) -> (-248.6977, 91.525) centre (-248.6977, 93.025) ccw
  arc A199 (-238.6977, 91.525) -> (-238.6977, 94.525) centre (-238.6977, 93.025) ccw
  line L303 (-248.6977, 94.525) -> (-238.6977, 94.525)
  line L304 (-248.6977, 91.525) -> (-243.6977, 91.525)
  line L305 (-238.6977, 91.525) -> (-243.6977, 91.525)
  arc A200 (-228.6977, 94.525) -> (-228.6977, 91.525) centre (-228.6977, 93.025) ccw
  arc A201 (-218.6977, 91.525) -> (-218.6977, 94.525) centre (-218.6977, 93.025) ccw
  line L306 (-228.6977, 94.525) -> (-218.6977, 94.525)
  line L307 (-228.6977, 91.525) -> (-223.6977, 91.525)
  line L308 (-218.6977, 91.525) -> (-223.6977, 91.525)
  arc A202 (-208.6977, 94.525) -> (-208.6977, 91.525) centre (-208.6977, 93.025) ccw
  arc A203 (-198.6977, 91.525) -> (-198.6977, 94.525) centre (-198.6977, 93.025) ccw
  line L309 (-208.6977, 94.525) -> (-198.6977, 94.525)
  line L310 (-208.6977, 91.525) -> (-203.6977, 91.525)
  line L311 (-198.6977, 91.525) -> (-203.6977, 91.525)
  arc A204 (-188.6977, 94.525) -> (-188.6977, 91.525) centre (-188.6977, 93.025) ccw
  arc A205 (-178.6977, 91.525) -> (-178.6977, 94.525) centre (-178.6977, 93.025) ccw
  line L312 (-188.6977, 94.525) -> (-178.6977, 94.525)
  line L313 (-188.6977, 91.525) -> (-183.6977, 91.525)
  line L314 (-178.6977, 91.525) -> (-183.6977, 91.525)
  arc A206 (-168.6977, 94.525) -> (-168.6977, 91.525) centre (-168.6977, 93.025) ccw
  arc A207 (-158.6977, 91.525) -> (-158.6977, 94.525) centre (-158.6977, 93.025) ccw
  line L315 (-168.6977, 94.525) -> (-158.6977, 94.525)
  line L316 (-168.6977, 91.525) -> (-163.6977, 91.525)
  line L317 (-158.6977, 91.525) -> (-163.6977, 91.525)
  arc A208 (-148.6977, 94.525) -> (-148.6977, 91.525) centre (-148.6977, 93.025) ccw
  arc A209 (-138.6977, 91.525) -> (-138.6977, 94.525) centre (-138.6977, 93.025) ccw
  line L318 (-148.6977, 94.525) -> (-138.6977, 94.525)
  line L319 (-148.6977, 91.525) -> (-143.6977, 91.525)
  line L320 (-138.6977, 91.525) -> (-143.6977, 91.525)
  arc A210 (-128.6977, 94.525) -> (-128.6977, 91.525) centre (-128.6977, 93.025) ccw
  arc A211 (-118.6977, 91.525) -> (-118.6977, 94.525) centre (-118.6977, 93.025) ccw
  line L321 (-128.6977, 94.525) -> (-118.6977, 94.525)
  line L322 (-128.6977, 91.525) -> (-123.6977, 91.525)
  line L323 (-118.6977, 91.525) -> (-123.6977, 91.525)
  arc A212 (-108.6977, 94.525) -> (-108.6977, 91.525) centre (-108.6977, 93.025) ccw
  arc A213 (-98.6977, 91.525) -> (-98.6977, 94.525) centre (-98.6977, 93.025) ccw
  line L324 (-108.6977, 94.525) -> (-98.6977, 94.525)
  line L325 (-108.6977, 91.525) -> (-103.6977, 91.525)
  line L326 (-98.6977, 91.525) -> (-103.6977, 91.525)
  arc A214 (-88.6977, 94.525) -> (-88.6977, 91.525) centre (-88.6977, 93.025) ccw
  arc A215 (-78.6977, 91.525) -> (-78.6977, 94.525) centre (-78.6977, 93.025) ccw
  line L327 (-88.6977, 94.525) -> (-78.6977, 94.525)
  line L328 (-88.6977, 91.525) -> (-83.6977, 91.525)
  line L329 (-78.6977, 91.525) -> (-83.6977, 91.525)
  arc A216 (-68.6977, 94.525) -> (-68.6977, 91.525) centre (-68.6977, 93.025) ccw
  arc A217 (-58.6977, 91.525) -> (-58.6977, 94.525) centre (-58.6977, 93.025) ccw
  line L330 (-68.6977, 94.525) -> (-58.6977, 94.525)
  line L331 (-68.6977, 91.525) -> (-63.6977, 91.525)
  line L332 (-58.6977, 91.525) -> (-63.6977, 91.525)
  arc A218 (-248.6977, 104.525) -> (-248.6977, 101.525) centre (-248.6977, 103.025) ccw
  arc A219 (-238.6977, 101.525) -> (-238.6977, 104.525) centre (-238.6977, 103.025) ccw
  line L333 (-248.6977, 104.525) -> (-238.6977, 104.525)
  line L334 (-248.6977, 101.525) -> (-243.6977, 101.525)
  line L335 (-238.6977, 101.525) -> (-243.6977, 101.525)
  arc A220 (-228.6977, 104.525) -> (-228.6977, 101.525) centre (-228.6977, 103.025) ccw
  arc A221 (-218.6977, 101.525) -> (-218.6977, 104.525) centre (-218.6977, 103.025) ccw
  line L336 (-228.6977, 104.525) -> (-218.6977, 104.525)
  line L337 (-228.6977, 101.525) -> (-223.6977, 101.525)
  line L338 (-218.6977, 101.525) -> (-223.6977, 101.525)
  arc A222 (-208.6977, 104.525) -> (-208.6977, 101.525) centre (-208.6977, 103.025) ccw
  arc A223 (-198.6977, 101.525) -> (-198.6977, 104.525) centre (-198.6977, 103.025) ccw
  line L339 (-208.6977, 104.525) -> (-198.6977, 104.525)
  line L340 (-208.6977, 101.525) -> (-203.6977, 101.525)
  line L341 (-198.6977, 101.525) -> (-203.6977, 101.525)
  arc A224 (-188.6977, 104.525) -> (-188.6977, 101.525) centre (-188.6977, 103.025) ccw
  arc A225 (-178.6977, 101.525) -> (-178.6977, 104.525) centre (-178.6977, 103.025) ccw
  line L342 (-188.6977, 104.525) -> (-178.6977, 104.525)
  line L343 (-188.6977, 101.525) -> (-183.6977, 101.525)
  line L344 (-178.6977, 101.525) -> (-183.6977, 101.525)
  arc A226 (-168.6977, 104.525) -> (-168.6977, 101.525) centre (-168.6977, 103.025) ccw
  arc A227 (-158.6977, 101.525) -> (-158.6977, 104.525) centre (-158.6977, 103.025) ccw
  line L345 (-168.6977, 104.525) -> (-158.6977, 104.525)
  line L346 (-168.6977, 101.525) -> (-163.6977, 101.525)
  line L347 (-158.6977, 101.525) -> (-163.6977, 101.525)
  arc A228 (-148.6977, 104.525) -> (-148.6977, 101.525) centre (-148.6977, 103.025) ccw
  arc A229 (-138.6977, 101.525) -> (-138.6977, 104.525) centre (-138.6977, 103.025) ccw
  line L348 (-148.6977, 104.525) -> (-138.6977, 104.525)
  line L349 (-148.6977, 101.525) -> (-143.6977, 101.525)
  line L350 (-138.6977, 101.525) -> (-143.6977, 101.525)
  arc A230 (-128.6977, 104.525) -> (-128.6977, 101.525) centre (-128.6977, 103.025) ccw
  arc A231 (-118.6977, 101.525) -> (-118.6977, 104.525) centre (-118.6977, 103.025) ccw
  line L351 (-128.6977, 104.525) -> (-118.6977, 104.525)
  line L352 (-128.6977, 101.525) -> (-123.6977, 101.525)
  line L353 (-118.6977, 101.525) -> (-123.6977, 101.525)
  arc A232 (-108.6977, 104.525) -> (-108.6977, 101.525) centre (-108.6977, 103.025) ccw
  arc A233 (-98.6977, 101.525) -> (-98.6977, 104.525) centre (-98.6977, 103.025) ccw
  line L354 (-108.6977, 104.525) -> (-98.6977, 104.525)
  line L355 (-108.6977, 101.525) -> (-103.6977, 101.525)
  line L356 (-98.6977, 101.525) -> (-103.6977, 101.525)
  arc A234 (-88.6977, 104.525) -> (-88.6977, 101.525) centre (-88.6977, 103.025) ccw
  arc A235 (-78.6977, 101.525) -> (-78.6977, 104.525) centre (-78.6977, 103.025) ccw
  line L357 (-88.6977, 104.525) -> (-78.6977, 104.525)
  line L358 (-88.6977, 101.525) -> (-83.6977, 101.525)
  line L359 (-78.6977, 101.525) -> (-83.6977, 101.525)
  arc A236 (-248.6977, 114.525) -> (-248.6977, 111.525) centre (-248.6977, 113.025) ccw
  arc A237 (-238.6977, 111.525) -> (-238.6977, 114.525) centre (-238.6977, 113.025) ccw
  line L360 (-248.6977, 114.525) -> (-238.6977, 114.525)
  line L361 (-248.6977, 111.525) -> (-243.6977, 111.525)
  line L362 (-238.6977, 111.525) -> (-243.6977, 111.525)
  arc A238 (-228.6977, 114.525) -> (-228.6977, 111.525) centre (-228.6977, 113.025) ccw
  arc A239 (-218.6977, 111.525) -> (-218.6977, 114.525) centre (-218.6977, 113.025) ccw
  line L363 (-228.6977, 114.525) -> (-218.6977, 114.525)
  line L364 (-228.6977, 111.525) -> (-223.6977, 111.525)
  line L365 (-218.6977, 111.525) -> (-223.6977, 111.525)
  arc A240 (-208.6977, 114.525) -> (-208.6977, 111.525) centre (-208.6977, 113.025) ccw
  arc A241 (-198.6977, 111.525) -> (-198.6977, 114.525) centre (-198.6977, 113.025) ccw
  line L366 (-208.6977, 114.525) -> (-198.6977, 114.525)
  line L367 (-208.6977, 111.525) -> (-203.6977, 111.525)
  line L368 (-198.6977, 111.525) -> (-203.6977, 111.525)
  arc A242 (-188.6977, 114.525) -> (-188.6977, 111.525) centre (-188.6977, 113.025) ccw
  arc A243 (-178.6977, 111.525) -> (-178.6977, 114.525) centre (-178.6977, 113.025) ccw
  line L369 (-188.6977, 114.525) -> (-178.6977, 114.525)
  line L370 (-188.6977, 111.525) -> (-183.6977, 111.525)
  line L371 (-178.6977, 111.525) -> (-183.6977, 111.525)
  arc A244 (-168.6977, 114.525) -> (-168.6977, 111.525) centre (-168.6977, 113.025) ccw
  arc A245 (-158.6977, 111.525) -> (-158.6977, 114.525) centre (-158.6977, 113.025) ccw
  line L372 (-168.6977, 114.525) -> (-158.6977, 114.525)
  line L373 (-168.6977, 111.525) -> (-163.6977, 111.525)
  line L374 (-158.6977, 111.525) -> (-163.6977, 111.525)
  arc A246 (-148.6977, 114.525) -> (-148.6977, 111.525) centre (-148.6977, 113.025) ccw
  arc A247 (-138.6977, 111.525) -> (-138.6977, 114.525) centre (-138.6977, 113.025) ccw
  line L375 (-148.6977, 114.525) -> (-138.6977, 114.525)
  line L376 (-148.6977, 111.525) -> (-143.6977, 111.525)
  line L377 (-138.6977, 111.525) -> (-143.6977, 111.525)
  arc A248 (-128.6977, 114.525) -> (-128.6977, 111.525) centre (-128.6977, 113.025) ccw
  arc A249 (-118.6977, 111.525) -> (-118.6977, 114.525) centre (-118.6977, 113.025) ccw
  line L378 (-128.6977, 114.525) -> (-118.6977, 114.525)
  line L379 (-128.6977, 111.525) -> (-123.6977, 111.525)
  line L380 (-118.6977, 111.525) -> (-123.6977, 111.525)
  arc A250 (-108.6977, 114.525) -> (-108.6977, 111.525) centre (-108.6977, 113.025) ccw
  arc A251 (-98.6977, 111.525) -> (-98.6977, 114.525) centre (-98.6977, 113.025) ccw
  line L381 (-108.6977, 114.525) -> (-98.6977, 114.525)
  line L382 (-108.6977, 111.525) -> (-103.6977, 111.525)
  line L383 (-98.6977, 111.525) -> (-103.6977, 111.525)
  arc A252 (-88.6977, 114.525) -> (-88.6977, 111.525) centre (-88.6977, 113.025) ccw
  arc A253 (-78.6977, 111.525) -> (-78.6977, 114.525) centre (-78.6977, 113.025) ccw
  line L384 (-88.6977, 114.525) -> (-78.6977, 114.525)
  line L385 (-88.6977, 111.525) -> (-83.6977, 111.525)
  line L386 (-78.6977, 111.525) -> (-83.6977, 111.525)
  arc A254 (-248.6977, 124.525) -> (-248.6977, 121.525) centre (-248.6977, 123.025) ccw
  arc A255 (-238.6977, 121.525) -> (-238.6977, 124.525) centre (-238.6977, 123.025) ccw
  line L387 (-248.6977, 124.525) -> (-238.6977, 124.525)
  line L388 (-248.6977, 121.525) -> (-243.6977, 121.525)
  line L389 (-238.6977, 121.525) -> (-243.6977, 121.525)
  arc A256 (-228.6977, 124.525) -> (-228.6977, 121.525) centre (-228.6977, 123.025) ccw
  arc A257 (-218.6977, 121.525) -> (-218.6977, 124.525) centre (-218.6977, 123.025) ccw
  line L390 (-228.6977, 124.525) -> (-218.6977, 124.525)
  line L391 (-228.6977, 121.525) -> (-223.6977, 121.525)
  line L392 (-218.6977, 121.525) -> (-223.6977, 121.525)
  arc A258 (-208.6977, 124.525) -> (-208.6977, 121.525) centre (-208.6977, 123.025) ccw
  arc A259 (-198.6977, 121.525) -> (-198.6977, 124.525) centre (-198.6977, 123.025) ccw
  line L393 (-208.6977, 124.525) -> (-198.6977, 124.525)
  line L394 (-208.6977, 121.525) -> (-203.6977, 121.525)
  line L395 (-198.6977, 121.525) -> (-203.6977, 121.525)
  arc A260 (-188.6977, 124.525) -> (-188.6977, 121.525) centre (-188.6977, 123.025) ccw
  arc A261 (-178.6977, 121.525) -> (-178.6977, 124.525) centre (-178.6977, 123.025) ccw
  line L396 (-188.6977, 124.525) -> (-178.6977, 124.525)
  line L397 (-188.6977, 121.525) -> (-183.6977, 121.525)
  line L398 (-178.6977, 121.525) -> (-183.6977, 121.525)
  arc A262 (-168.6977, 124.525) -> (-168.6977, 121.525) centre (-168.6977, 123.025) ccw
  arc A263 (-158.6977, 121.525) -> (-158.6977, 124.525) centre (-158.6977, 123.025) ccw
  line L399 (-168.6977, 124.525) -> (-158.6977, 124.525)
  line L400 (-168.6977, 121.525) -> (-163.6977, 121.525)
  line L401 (-158.6977, 121.525) -> (-163.6977, 121.525)
  arc A264 (-148.6977, 124.525) -> (-148.6977, 121.525) centre (-148.6977, 123.025) ccw
  arc A265 (-138.6977, 121.525) -> (-138.6977, 124.525) centre (-138.6977, 123.025) ccw
  line L402 (-148.6977, 124.525) -> (-138.6977, 124.525)
  line L403 (-148.6977, 121.525) -> (-143.6977, 121.525)
  line L404 (-138.6977, 121.525) -> (-143.6977, 121.525)
  arc A266 (-128.6977, 124.525) -> (-128.6977, 121.525) centre (-128.6977, 123.025) ccw
  arc A267 (-118.6977, 121.525) -> (-118.6977, 124.525) centre (-118.6977, 123.025) ccw
  line L405 (-128.6977, 124.525) -> (-118.6977, 124.525)
  line L406 (-128.6977, 121.525) -> (-123.6977, 121.525)
  line L407 (-118.6977, 121.525) -> (-123.6977, 121.525)
  arc A268 (-108.6977, 124.525) -> (-108.6977, 121.525) centre (-108.6977, 123.025) ccw
  arc A269 (-98.6977, 121.525) -> (-98.6977, 124.525) centre (-98.6977, 123.025) ccw
  line L408 (-108.6977, 124.525) -> (-98.6977, 124.525)
  line L409 (-108.6977, 121.525) -> (-103.6977, 121.525)
  line L410 (-98.6977, 121.525) -> (-103.6977, 121.525)
  arc A270 (-248.6977, 134.525) -> (-248.6977, 131.525) centre (-248.6977, 133.025) ccw
  arc A271 (-238.6977, 131.525) -> (-238.6977, 134.525) centre (-238.6977, 133.025) ccw
  line L411 (-248.6977, 134.525) -> (-238.6977, 134.525)
  line L412 (-248.6977, 131.525) -> (-243.6977, 131.525)
  line L413 (-238.6977, 131.525) -> (-243.6977, 131.525)
  arc A272 (-228.6977, 134.525) -> (-228.6977, 131.525) centre (-228.6977, 133.025) ccw
  arc A273 (-218.6977, 131.525) -> (-218.6977, 134.525) centre (-218.6977, 133.025) ccw
  line L414 (-228.6977, 134.525) -> (-218.6977, 134.525)
  line L415 (-228.6977, 131.525) -> (-223.6977, 131.525)
  line L416 (-218.6977, 131.525) -> (-223.6977, 131.525)
  arc A274 (-208.6977, 134.525) -> (-208.6977, 131.525) centre (-208.6977, 133.025) ccw
  arc A275 (-198.6977, 131.525) -> (-198.6977, 134.525) centre (-198.6977, 133.025) ccw
  line L417 (-208.6977, 134.525) -> (-198.6977, 134.525)
  line L418 (-208.6977, 131.525) -> (-203.6977, 131.525)
  line L419 (-198.6977, 131.525) -> (-203.6977, 131.525)
  arc A276 (-188.6977, 134.525) -> (-188.6977, 131.525) centre (-188.6977, 133.025) ccw
  arc A277 (-178.6977, 131.525) -> (-178.6977, 134.525) centre (-178.6977, 133.025) ccw
  line L420 (-188.6977, 134.525) -> (-178.6977, 134.525)
  line L421 (-188.6977, 131.525) -> (-183.6977, 131.525)
  line L422 (-178.6977, 131.525) -> (-183.6977, 131.525)
  arc A278 (-168.6977, 134.525) -> (-168.6977, 131.525) centre (-168.6977, 133.025) ccw
  arc A279 (-158.6977, 131.525) -> (-158.6977, 134.525) centre (-158.6977, 133.025) ccw
  line L423 (-168.6977, 134.525) -> (-158.6977, 134.525)
  line L424 (-168.6977, 131.525) -> (-163.6977, 131.525)
  line L425 (-158.6977, 131.525) -> (-163.6977, 131.525)
  arc A280 (-148.6977, 134.525) -> (-148.6977, 131.525) centre (-148.6977, 133.025) ccw
  arc A281 (-138.6977, 131.525) -> (-138.6977, 134.525) centre (-138.6977, 133.025) ccw
  line L426 (-148.6977, 134.525) -> (-138.6977, 134.525)
  line L427 (-148.6977, 131.525) -> (-143.6977, 131.525)
  line L428 (-138.6977, 131.525) -> (-143.6977, 131.525)
  arc A282 (-128.6977, 134.525) -> (-128.6977, 131.525) centre (-128.6977, 133.025) ccw
  arc A283 (-118.6977, 131.525) -> (-118.6977, 134.525) centre (-118.6977, 133.025) ccw
  line L429 (-128.6977, 134.525) -> (-118.6977, 134.525)
  line L430 (-128.6977, 131.525) -> (-123.6977, 131.525)
  line L431 (-118.6977, 131.525) -> (-123.6977, 131.525)
  arc A284 (-108.6977, 134.525) -> (-108.6977, 131.525) centre (-108.6977, 133.025) ccw
  arc A285 (-98.6977, 131.525) -> (-98.6977, 134.525) centre (-98.6977, 133.025) ccw
  line L432 (-108.6977, 134.525) -> (-98.6977, 134.525)
  line L433 (-108.6977, 131.525) -> (-103.6977, 131.525)
  line L434 (-98.6977, 131.525) -> (-103.6977, 131.525)
  arc A286 (-228.6977, 144.525) -> (-228.6977, 141.525) centre (-228.6977, 143.025) ccw
  arc A287 (-218.6977, 141.525) -> (-218.6977, 144.525) centre (-218.6977, 143.025) ccw
  line L435 (-228.6977, 144.525) -> (-218.6977, 144.525)
  line L436 (-228.6977, 141.525) -> (-223.6977, 141.525)
  line L437 (-218.6977, 141.525) -> (-223.6977, 141.525)
  arc A288 (-208.6977, 144.525) -> (-208.6977, 141.525) centre (-208.6977, 143.025) ccw
  arc A289 (-198.6977, 141.525) -> (-198.6977, 144.525) centre (-198.6977, 143.025) ccw
  line L438 (-208.6977, 144.525) -> (-198.6977, 144.525)
  line L439 (-208.6977, 141.525) -> (-203.6977, 141.525)
  line L440 (-198.6977, 141.525) -> (-203.6977, 141.525)
  arc A290 (-188.6977, 144.525) -> (-188.6977, 141.525) centre (-188.6977, 143.025) ccw
  arc A291 (-178.6977, 141.525) -> (-178.6977, 144.525) centre (-178.6977, 143.025) ccw
  line L441 (-188.6977, 144.525) -> (-178.6977, 144.525)
  line L442 (-188.6977, 141.525) -> (-183.6977, 141.525)
  line L443 (-178.6977, 141.525) -> (-183.6977, 141.525)
  arc A292 (-168.6977, 144.525) -> (-168.6977, 141.525) centre (-168.6977, 143.025) ccw
  arc A293 (-158.6977, 141.525) -> (-158.6977, 144.525) centre (-158.6977, 143.025) ccw
  line L444 (-168.6977, 144.525) -> (-158.6977, 144.525)
  line L445 (-168.6977, 141.525) -> (-163.6977, 141.525)
  line L446 (-158.6977, 141.525) -> (-163.6977, 141.525)